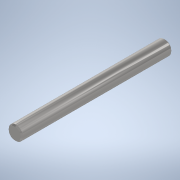
# Autodesk Inventor part: NASA-20-HUB-SHFT-01
Saved by Autodesk Inventor 2020 (Build 240168000, 168)
## iProperties
Created: 2019-09-22
Part Number: NASA-20-HUB-SHFT-01
Material: Steel, Alloy
Document SubType Name: Modeling
Designer: Rick Szalay
Density: 7.73 g/cm^3
Appearance: Semi-Polished
Description: SHAFT 6MM
Author: Rick Szalay
Autodesk Inventor part; units mm, degrees
ref_plane "YZ Plane" through (0, 0, 0) normal (1, 0, 0) x (0, 1, 0)
ref_plane "XZ Plane" through (0, 0, 0) normal (0, 1, 0) x (-1, 0, 0)
ref_plane "XY Plane" through (0, 0, 0) normal (0, 0, 1) x (1, 0, 0)
sketch "Sketch1" plane through (0, 0, 0) normal (0, 0, 1) x (1, 0, 0)
  circle A0 centre (0, 0) radius 3
  dimension "d0" = 6
  constraints: 1 centre point, 1 coincident
  measures "d0" diameter of A0
extrude "Extrusion1" add sketch "Sketch1" along normal mid plane 63.5
chamfer "Chamfer1" distance 0.5 angle 45 2 edges at (-3, 0, 31.75) (-3, 0, -31.75)
body "Solid1"
